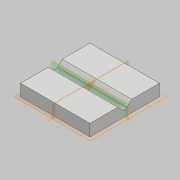
# Autodesk Inventor part: Placa - Grieta
Saved by Autodesk Inventor 2017 (Build 210142000, 142)
## iProperties
Part Number: Placa - Grieta
Material: Genérico
Document SubType Name: Modeling
Designer: franc
Density: 1 g/cm^3
Appearance: Valor por defecto
Author: franc
Autodesk Inventor part; units mm, degrees
sketch "Boceto1" plane through (0, 0, 0) normal (0, 0, 1) x (1, 0, 0)
  line L0 (-75, 75) -> (75, 75)
  line L1 (75, 75) -> (75, -75)
  line L2 (75, -75) -> (-75, -75)
  line L3 (-75, -75) -> (-75, 75)
  line L4 (-75, 75) -> (75, -75) construction
  line L5 (75, 75) -> (-75, -75) construction
  point P0 (0, 0)
  dimension "d0" = 150
  dimension "d1" = 150
  constraints: 12 end point, 2 midpoint, 2 parallel, 1 horizontal, 1 perpendicular
  measures "d0" distance of L1.end L2.end
  measures "d1" distance of L0.end L1.end
extrude "Extrusión1" add sketch "Boceto1" along normal blind 25.4
sketch "Boceto2" plane through (75, -75, 0) normal (1, 0, 0) x (0, 0, -1)
  line L0 (-25.4, 150) -> (-25.4, 0) projected
  line L1 (-25.4, 0) -> (-25.4, 150) projected
  line L2 (-25.4, 75) -> (-25.4, 60)
  line L3 (-25.4, 75) -> (-10.4, 75)
  line L4 (-10.4, 75) -> (-25.4, 60)
  line L5 (-25.4, 75) -> (-25.4, 90)
  line L6 (-25.4, 90) -> (-10.4, 75)
  point P0 (0, 75)
  dimension "d6" = 15
  dimension "d7" = 15
  dimension "d9" = 15
  constraints: 10 end point, 2 point on line, 1 midpoint, 1 perpendicular
  measures "d6" distance of L2.start L2.end
  measures "d7" distance of L2.start L3.end
  measures "d9" distance of L2.start L5.end
extrude "Extrusión2" cut sketch "Boceto2" against normal blind 165.25
fillet "Empalme1" radius 7 1 edges at (0, 0, 10.4)
